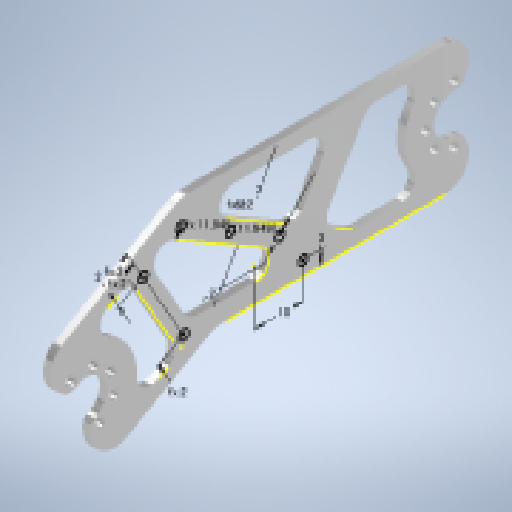
# Autodesk Inventor part: leg_upper_outside
Saved by Autodesk Inventor 2024.1 (Build 281209000, 209)
## iProperties
Created: 2023-08-04
Part Number: leg_upper_outside
Material: アルミニウム 6061
Document SubType Name: Modeling
Designer: hibik
Density: 2.7 g/cm^3
Appearance: アルミニウム - フラット
Author: hibik
Autodesk Inventor part; units mm, degrees
ref_plane "YZ Plane" through (0, 0, 0) normal (1, 0, 0) x (0, 1, 0)
ref_plane "XZ Plane" through (0, 0, 0) normal (0, 1, 0) x (-1, 0, 0)
ref_plane "XY Plane" through (0, 0, 0) normal (0, 0, 1) x (1, 0, 0)
sketch "スケッチ1" plane through (0, 0, 0) normal (1, 0, 0) x (0, 1, 0)
  line L0 (27, 0) -> (0, 0)
  line L1 (0, 0) -> (0, -65.872265)
  line L2 (0, -65.872265) -> (27, -65.872265)
  line L3 (27, -65.872265) -> (27, 0)
  line L4 (27, 0) -> (7.296343, 34.127735)
  line L5 (7.296343, 34.127735) -> (-16.086343, 20.627735)
  line L6 (-16.086343, 20.627735) -> (0, -7.234628)
  line L7 (0, 19.765372) -> (-4.395, 27.377735)
  circle A0 centre (0, 19.765372) radius 4.25
  circle A1 centre (13.5, -57.082265) radius 4.25
  line L8 (13.5, -65.872265) -> (13.5, -57.082265)
  circle A2 centre (0, 19.765372) radius 13.5
  circle A3 centre (13.5, -57.082265) radius 13.5
  line L9 (5.064542, 0) -> (22.68082, 0)
  circle A4 centre (0, 19.765372) radius 6
  circle A5 centre (13.5, -57.082265) radius 6
  circle A6 centre (-3, 24.961524) radius 1
  circle A7 centre (-5.795555, 21.318286) radius 1
  circle A8 centre (-5.196152, 16.765372) radius 1
  circle A9 centre (-1.552914, 13.969817) radius 1
  circle A10 centre (3, 14.569219) radius 1
  circle A11 centre (5.795555, 18.212458) radius 1
  circle A12 centre (13.5, -63.082265) radius 1
  circle A13 centre (17.742641, -61.324906) radius 1
  circle A14 centre (19.5, -57.082265) radius 1
  circle A15 centre (17.742641, -52.839624) radius 1
  circle A16 centre (13.5, -51.082265) radius 1
  circle A17 centre (9.257359, -52.839624) radius 1
  circle A18 centre (7.5, -57.082265) radius 1
  circle A19 centre (9.257359, -61.324906) radius 1
  circle A20 centre (5.196152, 22.765372) radius 1
  circle A21 centre (1.552914, 25.560927) radius 1
  line L10 (0, 19.765372) -> (8.218279, 30.475642)
  line L11 (0, 19.765372) -> (-13.384506, 18.003268)
  line L12 (8.218279, 30.475642) -> (-13.384506, 18.003268) construction
  line L13 (13.5, -57.082265) -> (25.972374, -62.248491)
  line L14 (13.5, -57.082265) -> (1.027626, -62.248491)
  point P0 (-11.691343, 13.015372)
  point P1 (0, -57.082265)
  point P2 (27, -57.082265)
  point P3 (11.691343, 26.515372)
  point P4 (2.587236, 23.137124)
  point P5 (-4.213641, 19.210635)
  point P6 (9.573512, -58.708669)
  point P7 (17.426488, -58.708669)
  dimension "d79" = 12
  dimension "d80" = 12
  dimension "d0" = 27
  dimension "d10" = 150
  dimension "d11" = 27
  dimension "d13" = 8.79
  dimension "d14" = 100
  dimension "d15" = 8.79
  dimension "d16" = 8.5
  dimension "d81" = 2
  dimension "d84" = 360
  dimension "d86" = 2
  dimension "d89" = 360
  dimension "d100" = 39.40731
  dimension "d102" = 2.2961
  dimension "d103" = 2.2961
  dimension "d105" = 2.2961
  dimension "d106" = 2.2961
  constraints: 30 end point, 20 centre point, 7 coincident, 4 perpendicular, 4 point on circle, 4 point on line, 2 midpoint, 2 parallel, 2 tangent, 2 vertical alignment, 1 equal radius, 1 horizontal, 1 vertical, 40 other
  measures "d0" distance of L1.end L2.end
  measures "d10" angle of L3 L4
  measures "d11" distance between parallel lines of L6 L4
  measures "d13" distance from line of L5 L7.start
  measures "d14" distance from line of L2 L4.end
  measures "d15" distance of L8.start point (13.5, -57.082)
  measures "d16" diameter of A0
  measures "d81" diameter of A6
  measures "d86" diameter of A12
  measures "d100" distance from line of L0.start L5
  measures "d102" distance from line of A20.centre L10
  measures "d103" distance from line of L10 A21.centre
  measures "d105" distance from line of A14.centre L13
  measures "d106" distance from line of L14 A18.centre
sketch "スケッチ1 outline for 押し出し1" plane through (0, 0, 0) normal (1, 0, 0) x (0, 1, 0)
  line L0 (17.426488, -58.708669) -> (25.972374, -62.248491)
  arc A0 (9.573512, -58.708669) -> (17.426488, -58.708669) centre (13.5, -57.082265) cw
  arc A1 (25.972374, -62.248491) -> (27, -57.082265) centre (13.5, -57.082265) ccw
  line L1 (1.027626, -62.248491) -> (9.573512, -58.708669)
  line L2 (27, -57.082265) -> (27, 0)
  arc A2 (0, -57.082265) -> (1.027626, -62.248491) centre (13.5, -57.082265) ccw
  line L3 (27, 0) -> (11.691343, 26.515372)
  line L4 (0, -7.234628) -> (0, -57.082265)
  arc A3 (11.691343, 26.515372) -> (8.218279, 30.475642) centre (0, 19.765372) ccw
  line L5 (-11.691343, 13.015372) -> (0, -7.234628)
  line L6 (8.218279, 30.475642) -> (2.587236, 23.137124)
  arc A4 (-13.384506, 18.003268) -> (-11.691343, 13.015372) centre (0, 19.765372) ccw
  arc A5 (2.587236, 23.137124) -> (-4.213641, 19.210635) centre (0, 19.765372) cw
  line L7 (-4.213641, 19.210635) -> (-13.384506, 18.003268)
  circle A6 centre (7.5, -57.082265) radius 1
  circle A7 centre (9.257359, -52.839624) radius 1
  circle A8 centre (13.5, -51.082265) radius 1
  circle A9 centre (19.5, -57.082265) radius 1
  circle A10 centre (17.742641, -52.839624) radius 1
  circle A11 centre (-5.196152, 16.765372) radius 1
  circle A12 centre (-1.552914, 13.969817) radius 1
  circle A13 centre (3, 14.569219) radius 1
  circle A14 centre (5.795555, 18.212458) radius 1
  circle A15 centre (5.196152, 22.765372) radius 1
extrude "押し出し1" add sketch "スケッチ1 outline for 押し出し1" along normal blind 1.5
fillet "フィレット1" radius 8 2 edges at (0.75, 27, 0) (0.75, 0, -7.2346)
fillet "フィレット6" radius 5 4 edges at (0.75, 1.0276, -62.2485) (0.75, 25.9724, -62.2485) (0.75, -13.3845, 18.0033) (0.75, 8.2183, 30.4756)
fillet "フィレット7" radius 2 4 edges at (0.75, 2.5872, 23.1371) (0.75, -4.2136, 19.2106) (0.75, 9.5735, -58.7087) (0.75, 17.4265, -58.7087)
sketch "スケッチ9" plane through (1.5, 0, 0) normal (1, 0, 0) x (0, 0, -1)
  line L0 (0.849789, 23.449174) -> (-2.650211, 25.4699)
  arc A0 (9.334617, -0.000119) -> (5.378222, -1.071797) centre (9.378222, -8) ccw
  line L1 (1.274047, -3.441343) -> (5.378222, -1.071797)
  line L2 (-12.225953, 19.941343) -> (1.274047, -3.441343)
  line L3 (-2.650211, 25.4699) -> (-12.225953, 19.941343)
  line L4 (55.191119, 27) -> (2.143594, 27)
  line L5 (-5.300421, 27) -> (41.464951, 0)
  line L6 (9.378222, 0) -> (55.191119, 0)
  line L7 (-0.104269, 24) -> (57.082265, 24)
  arc A1 (57.366673, 17.740473) -> (57.366673, 9.259527) centre (57.082265, 13.5) ccw
  circle A2 centre (57.082265, 13.5) radius 10.5
  line L8 (57.082265, 3) -> (36.268798, 3)
  line L9 (24.144443, 10) -> (32.227346, 24)
  line L10 (39.15555, 24) -> (29.340595, 7)
  line L11 (-6.761851, 18.477241) -> (-2.650211, 20.851098)
  line L12 (-2.650211, 20.851098) -> (26.536748, 4)
  line L13 (26.536748, 4) -> (1.596588, 4)
  line L14 (1.596588, 4) -> (-6.761851, 18.477241)
  line L15 (-1.856406, 25.928203) -> (-24.877592, 12.636916)
  arc A3 (-17.89144, -3.814561) -> (-22.131913, 3.530153) centre (-19.765372, 0) ccw
  circle A4 centre (-19.765372, 0) radius 10.5
  line L16 (-25.015372, 9.093267) -> (-10.725953, 17.343267)
  line L17 (-14.515372, -9.093267) -> (-0.225953, -0.843267)
  arc A5 (0.730563, 5.5) -> (3.328639, 4) centre (3.328639, 7) ccw
  line L18 (3.328639, 4) -> (9.334617, 4)
  arc A6 (-1.150211, 19.985073) -> (-4.150211, 19.985073) centre (-2.650211, 17.386996) ccw
  line L19 (-4.150211, 19.985073) -> (-4.163775, 19.977241)
  arc A7 (-4.163775, 19.977241) -> (-5.261851, 15.879165) centre (-2.663775, 17.379165) ccw
  line L20 (-5.261851, 15.879165) -> (0.730563, 5.5)
  line L21 (9.334617, -0.000119) -> (9.334617, 4)
  line L22 (-1.150211, 19.985073) -> (0.849789, 23.449174)
  circle A8 centre (-6.895826, 20.709292) radius 0.8
  circle A9 centre (5.506098, 2) radius 0.8
  circle A10 centre (-7.993902, 16.611216) radius 0.8
  circle A11 centre (0.506098, 1.888784) radius 0.8
  point P0 (0, 0)
  point P1 (36.073935, 0)
  point P2 (15.340595, 4)
  point P3 (16.840595, 9.598076)
  point P4 (-2.650211, 17.386996)
  dimension "d109" = 0
  dimension "d110" = 3
  dimension "d111" = 6
  dimension "d112" = 8
  dimension "d118" = 4
  dimension "d119" = 4
  dimension "d120" = 4
  constraints: 22 end point, 10 point on line, 5 parallel, 4 point on circle, 4 tangent, 3 horizontal, 2 centre point, 2 coincident, 2 perpendicular, 1 collinear, 1 equal radius
  measures "d109" distance between parallel lines of L5 L0
  measures "d110" distance between parallel lines of L4 L7
  measures "d111" distance between parallel lines of L10 L9
  measures "d112" distance from line of L8.end L10
  measures "d118" distance between parallel lines of L0 L12
  measures "d119" distance between parallel lines of L11 L3
  measures "d120" distance between parallel lines of L2 L14
sketch "スケッチ9 outline for 押し出し10" plane through (1.5, 0, 0) normal (1, 0, 0) x (0, 0, -1)
  line L0 (39.15555, 24) -> (29.340595, 7)
  line L1 (57.082265, 24) -> (39.15555, 24)
  arc A0 (57.082265, 3) -> (57.082265, 24) centre (57.082265, 13.5) cw
  line L2 (36.268798, 3) -> (57.082265, 3)
  line L3 (29.340595, 7) -> (36.268798, 3)
  line L4 (24.144443, 10) -> (32.227346, 24)
  line L5 (-0.104269, 24) -> (24.144443, 10)
  line L6 (32.227346, 24) -> (-0.104269, 24)
  line L7 (-14.515372, -9.093267) -> (-0.225953, -0.843267)
  arc A1 (-25.015372, 9.093267) -> (-14.515372, -9.093267) centre (-19.765372, 0) cw
  line L8 (-10.725953, 17.343267) -> (-25.015372, 9.093267)
  line L9 (-0.225953, -0.843267) -> (-10.725953, 17.343267)
  line L10 (-6.761851, 18.477241) -> (1.596588, 4)
  line L11 (-2.650211, 20.851098) -> (-6.761851, 18.477241)
  line L12 (26.536748, 4) -> (-2.650211, 20.851098)
  line L13 (1.596588, 4) -> (26.536748, 4)
extrude "押し出し10" cut sketch "スケッチ9 outline for 押し出し10" against normal through all
fillet "フィレット8" radius 3 16 edges at (0.75, 24, -57.0823) (0.75, 7, -29.3406) (0.75, 24, -39.1555) (0.75, 3, -36.2688) (0.75, 24, -32.2273) (0.75, 10, -24.1444) (0.75, 24, 0.1043) (0.75, 3, -57.0823) (0.75, 20.8511, 2.6502) (0.75, 18.4772, 6.7619) (0.75, 4, -1.5966) (0.75, 4, -26.5367) (0.75, 17.3433, 10.726) (0.75, -0.8433, 0.226) (0.75, -9.0933, 14.5154) (0.75, 9.0933, 25.0154)
sketch "スケッチ10" plane through (1.5, 0, 0) normal (1, 0, 0) x (0, 0, -1)
  circle A0 centre (20.546367, 9.767949) radius 1
  line L0 (21.546367, 11.5) -> (9.591884, 18.401924)
  circle A1 centre (-0.150211, 21.717124) radius 1
  circle A2 centre (0.506098, 1.888784) radius 1
  circle A3 centre (-7.993902, 16.611216) radius 1
  circle A4 centre (25.340595, 3) radius 1
  line L1 (35.572646, 3.401924) -> (31.938671, 5.5)
  arc A5 (15.340595, 4) -> (16.840595, 9.598076) centre (15.340595, 7) ccw
  line L2 (9.378222, 0) -> (55.191119, 0)
  line L3 (-1.150211, 19.985073) -> (16.840595, 9.598076)
  line L4 (-15.294261, 14.705753) -> (-13.324029, 15.843267)
  line L5 (-2.824029, -2.343267) -> (-4.794261, -3.480781)
  line L6 (-9.225953, 14.745191) -> (-1.725953, 1.754809)
  line L7 (21.546367, 11.5) -> (20.546367, 9.767949)
  line L8 (-1.150211, 19.985073) -> (-0.150211, 21.717124)
  circle A6 centre (10.198078, 15.742536) radius 1
  circle A7 centre (5.506098, 2) radius 1
  circle A8 centre (-6.895826, 20.709292) radius 1
  line L9 (-1.856406, 25.928203) -> (-24.877592, 12.636916)
  point P0 (0, 0)
  dimension "d121" = 2
  dimension "d122" = 2
  dimension "d124" = 2
  dimension "d128" = 3
  dimension "d129" = 2
  dimension "d130" = 2
  dimension "d131" = 2
  dimension "d132" = 2
  dimension "d133" = 10
  dimension "d134" = 2
  dimension "d135" = 11.94917
  dimension "d136" = 11.94917
  dimension "d137" = 2
  dimension "d138" = 5
  dimension "d139" = 2
  dimension "d140" = 5
  constraints: 8 centre point, 7 equal radius, 4 end point, 2 perpendicular
  measures "d121" diameter of A0
  measures "d122" distance from line of L0 L7.end
  measures "d124" distance from line of L0 L8.end
  measures "d128" distance from line of L2 A4.centre
  measures "d129" distance from line of L4 A3.centre
  measures "d130" distance from line of L5 A2.centre
  measures "d131" distance from line of L6 A3.centre
  measures "d132" distance from line of A2.centre L6
  measures "d133" horizontal distance of A5.centre A4.centre
  measures "d134" distance from line of L0 A6.centre
  measures "d135" distance from line of A6.centre L8
  measures "d136" distance from line of A6.centre L7
  measures "d137" distance from line of L2 A7.centre
  measures "d138" horizontal distance of A2.centre A7.centre
  measures "d139" distance from line of L9 A8.centre
  measures "d140" distance from line of L6 A8.centre
sketch "スケッチ10 outline for 押し出し11" plane through (1.5, 0, 0) normal (1, 0, 0) x (0, 0, -1)
  circle A0 centre (20.546367, 9.767949) radius 1
  circle A1 centre (10.198078, 15.742536) radius 1
  circle A2 centre (-7.993902, 16.611216) radius 1
  circle A3 centre (0.506098, 1.888784) radius 1
  circle A4 centre (5.506098, 2) radius 1
  circle A5 centre (25.340595, 3) radius 1
  circle A6 centre (-6.895826, 20.709292) radius 1
extrude "押し出し11" cut sketch "スケッチ10 outline for 押し出し11" against normal through all
